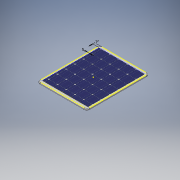
# Autodesk Inventor part: Solar Panel
Saved by Autodesk Inventor 2019 (Build 230136000, 136)
## iProperties
Created: 2020-02-21
Part Number: Solar Panel
Material: Generic
Document SubType Name: Modeling
Designer: gfb14170
Density: 1 g/cm^3
Appearance: Default
Author: gfb14170
Autodesk Inventor part; units mm, degrees
ref_plane "YZ Plane" through (0, 0, 0) normal (1, 0, 0) x (0, 1, 0)
ref_plane "XZ Plane" through (0, 0, 0) normal (0, 1, 0) x (-1, 0, 0)
ref_plane "XY Plane" through (0, 0, 0) normal (0, 0, 1) x (1, 0, 0)
sketch "Sketch1" plane through (0, 0, 0) normal (0, 1, 0) x (-1, 0, 0)
  line L0 (87.5, 110) -> (-87.5, 110)
  line L1 (-87.5, 110) -> (-87.5, -110)
  line L2 (-87.5, -110) -> (87.5, -110)
  line L3 (87.5, -110) -> (87.5, 110)
  point P0 (0, 0)
  dimension "d0" = 110
  dimension "d1" = 110
  dimension "d2" = 87.5
  dimension "d3" = 87.5
  constraints: 8 end point, 2 parallel, 1 horizontal, 1 perpendicular
  measures "d0" distance from line of L0 point (0, 0)
  measures "d1" distance from line of point (0, 0) L2
  measures "d2" distance from line of point (0, 0) L3
  measures "d3" distance from line of L1 point (0, 0)
extrude "Extrusion1" add sketch "Sketch1" along normal blind 4.5
fillet "Fillet1" radius 10 4 edges at (-87.5, 2.25, 110) (-87.5, 2.25, -110) (87.5, 2.25, -110) (87.5, 2.25, 110)
fillet "Fillet2" radius 2 8 edges at (-84.5711, 4.5, 107.0711) (0, 4.5, 110) (84.5711, 4.5, 107.0711) (87.5, 4.5, 0) (84.5711, 4.5, -107.0711) (0, 4.5, -110) (-84.5711, 4.5, -107.0711) (-87.5, 4.5, 0)
sketch "Sketch2" plane through (0, 0, 0) normal (0, -1, 0) x (1, 0, 0)
  circle A0 centre (-80.5, -103) radius 1
  line L0 (77.5, -110) -> (-77.5, -110) projected
  line L1 (-87.5, -100) -> (-87.5, 100) projected
  circle A1 centre (79.5, -103) radius 1
  circle A2 centre (-80.5, 102) radius 1
  circle A3 centre (79.5, 102) radius 1
  point P0 (0, 0)
  dimension "d8" = 7
  dimension "d9" = 7
  dimension "d10" = 2
  dimension "d13" = 160
  dimension "d16" = 205
  constraints: 4 centre point, 1 horizontal, 1 vertical, 6 other
  measures "d8" distance from line of L0 A0.centre
  measures "d9" distance from line of L1 A0.centre
  measures "d10" diameter of A0
  measures "d13" distance of A0.centre A1.centre
  measures "d16" distance of A0.centre A2.centre
extrude "Extrusion2" add sketch "Sketch2" along normal blind 5
sketch "Sketch3" plane through (0, 4.5, 0) normal (0, 1, 0) x (1, 0, 0)
  line L0 (-77.5, 108) -> (77.5, 108) projected
  line L1 (85.5, 100) -> (85.5, -100) projected
  line L2 (77.5, -108) -> (-77.5, -108) projected
  line L3 (-85.5, -100) -> (-85.5, 100) projected
  line L4 (-80.5, 101) -> (81.8602, 101) construction
  line L5 (81.8602, 101) -> (81.8602, -100.4389) construction
  line L6 (81.8602, -100.4389) -> (-80.5, -100.4389) construction
  line L7 (-80.5, -100.4389) -> (-80.5, 101) construction
  point P0 (0, 0)
  dimension "d98" = 7
  dimension "d99" = 5
  constraints: 2 other
  measures "d98" distance between parallel lines of L0 L4
  measures "d99" distance between parallel lines of L7 L3
equation "\"d1\" = d0"
equation "\"d3\" = d2"
body "Solid1"
